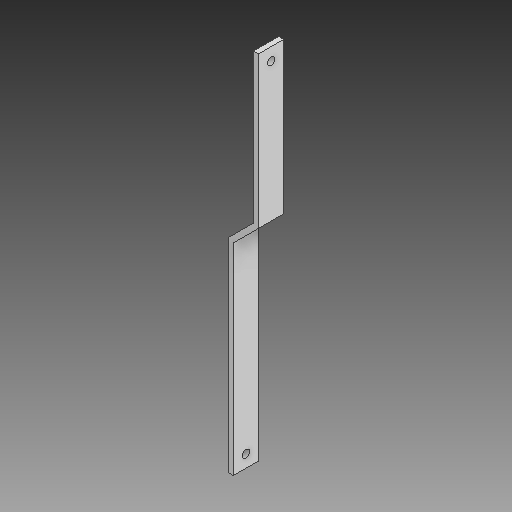
# Autodesk Inventor part: Gestänge
Saved by Autodesk Inventor 2021 (Build 250183000, 183)
## iProperties
Created: 2022-03-14
Part Number: Gestänge
Material: Generisch
Document SubType Name: Modeling
Designer: lukas
Density: 1 g/cm^3
Appearance: Vorgabe
Stock Number: Gestänge
Author: lukas
Autodesk Inventor part; units mm, degrees
ref_plane "YZ Plane" through (0, 0, 0) normal (1, 0, 0) x (0, 1, 0)
ref_plane "XZ Plane" through (0, 0, 0) normal (0, 1, 0) x (-1, 0, 0)
ref_plane "XY Plane" through (0, 0, 0) normal (0, 0, 1) x (1, 0, 0)
sketch "Skizze1" plane through (0, 0, 0) normal (0, 0, 1) x (1, 0, 0)
  line L0 (-14.4, 0) -> (2.4, 0) projected
  line L1 (0, -68.8373) -> (0, 141.1627) projected
  line L2 (-10, -38.8373) -> (-10, 41.1627)
  line L3 (-10, 41.1627) -> (0, 51.1627)
  line L4 (0, 51.1627) -> (0, 111.1627)
  line L5 (-10, -38.8373) -> (-12, -38.8373)
  line L6 (-12, -38.8373) -> (-12, 41.9912)
  line L7 (-2, 51.9912) -> (-12, 41.9912)
  line L8 (-2, 111.1627) -> (0, 111.1627)
  line L9 (-2, 111.1627) -> (-2, 51.9912)
  point P0 (0, 0)
  dimension "d0" = 80
  dimension "d2" = 60
  dimension "d5" = 2
  dimension "d6" = 2
  dimension "d7" = 2
  dimension "d20" = 10
  dimension "d22" = 150
  constraints: 16 end point, 3 parallel, 2 horizontal, 2 point on line, 2 vertical
  measures "d0" distance of L2.start L2.end
  measures "d2" distance of L3.end L4.end
  measures "d5" distance between parallel lines of L2 L6
  measures "d6" distance between parallel lines of L3 L7
  measures "d7" distance between parallel lines of L4 L9
  measures "d20" distance between parallel lines of L1 L2
  measures "d22" distance between parallel lines of L8 L5
extrude "Extrusion1" add sketch "Skizze1" against normal blind 10 contours L6 L7 L9 L8 L1 L3 L2 L0 | L0 L2 L5 L6
sketch "Skizze2" plane through (-12, -38.8373, 0) normal (-1, 0, 0) x (0, 0, 1)
  line L0 (0, 80.8284) -> (0, 0) projected
  line L1 (0, 0) -> (-10, 0) projected
  circle A0 centre (-5, 5) radius 1.5
  point P0 (0, 38.8373)
  dimension "d10" = 5
  dimension "d11" = 5
  dimension "d12" = 3
  constraints: 1 centre point, 1 coincident
  measures "d10" distance from line of point (-5, 5) L0
  measures "d11" distance from line of point (-5, 5) L1
  measures "d12" diameter of A0
extrude "Extrusion2" cut sketch "Skizze2" against normal blind 5
sketch "Skizze3" plane through (-2, 51.9912, 0) normal (-1, 0, 0) x (0, 0, 1)
  line L0 (-10, 0) -> (-10, 59.1716) projected
  line L1 (0, 59.1716) -> (-10, 59.1716) projected
  circle A0 centre (-5, 54.1716) radius 1.5
  point P0 (0, -51.9912)
  dimension "d15" = 5
  dimension "d16" = 5
  dimension "d17" = 3
  constraints: 1 centre point, 1 coincident
  measures "d15" distance from line of L0 point (-5, 54.172)
  measures "d16" distance from line of point (-5, 54.172) L1
  measures "d17" diameter of A0
extrude "Extrusion3" cut sketch "Skizze3" against normal blind 5
